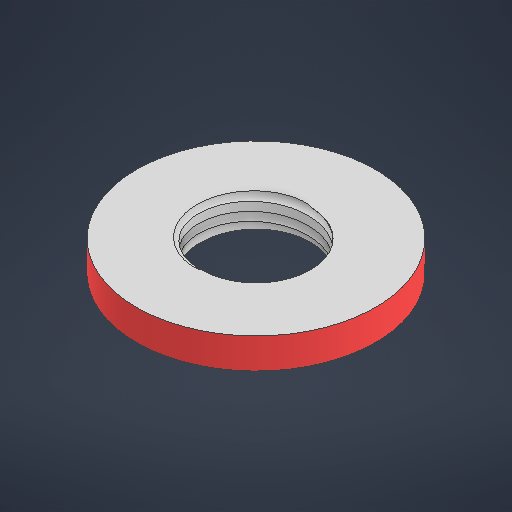
# Autodesk Inventor part: screwspoolv2
Saved by Autodesk Inventor 2027 (Build 310192060, 192F)
## iProperties
Created: 2026-06-22
Part Number: screwspoolv2
Material: Generic
Document SubType Name: Modeling
Designer: beave
Density: 1 g/cm^3
Appearance: Default
Author: beave
Autodesk Inventor part; units mm, degrees
ref_plane "YZ Plane" through (0, 0, 0) normal (1, 0, 0) x (0, 1, 0)
ref_plane "XZ Plane" through (0, 0, 0) normal (0, 1, 0) x (-1, 0, 0)
ref_plane "XY Plane" through (0, 0, 0) normal (0, 0, 1) x (1, 0, 0)
sketch "Sketch1" plane through (0, 0, 0) normal (0, 1, 0) x (-1, 0, 0)
  circle A0 centre (0, 0) radius 27.5
  dimension "d0" = 55
  constraints: 1 centre point, 1 coincident
  measures "d0" diameter of A0
extrude "Extrusion1" add sketch "Sketch1" along normal blind 7
sketch "Sketch2" plane through (0, 7, 0) normal (0, 1, 0) x (1, 0, 0)
  circle A0 centre (0, 0) radius 27.5 projected
  constraints: 2 coincident
hole "Hole1" at (0, 7, 0) direction (0, -1, 0) diameter 25.1 end through all
sketch "Sketch9" plane through (0, 0, 0) normal (0, 0, 1) x (1, 0, 0)
  circle A0 centre (-12.55, -1) radius 1
  line L0 (12.55, 0) -> (-12.55, 0) projected
  point P0 (0, 0)
  dimension "d52" = 2
  dimension "d53" = 1
  constraints: 1 centre point
  measures "d52" diameter of A0
  measures "d53" distance from line of L0 A0.centre
coil "Coil4" sketch "Sketch9" operation cut axis through (0, -10, 0) along (0, 1, 0) pitch 4 turns 2.75 hand right
body "Solid1"
